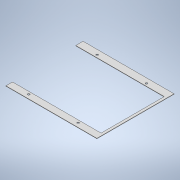
# Autodesk Inventor part: mainBody
Saved by Autodesk Inventor 2020.3 (Build 243373000, 373)
## iProperties
Created: 2021-03-06
Part Number: mainBody
Material: Generic
Document SubType Name: Modeling
Designer: allofus
Density: 1 g/cm^3
Appearance: Default
Author: allofus
Autodesk Inventor part; units mm, degrees
ref_plane "YZ Plane" through (0, 0, 0) normal (1, 0, 0) x (0, 1, 0)
ref_plane "XZ Plane" through (0, 0, 0) normal (0, 1, 0) x (-1, 0, 0)
ref_plane "XY Plane" through (0, 0, 0) normal (0, 0, 1) x (1, 0, 0)
sketch "Sketch1" plane through (0, 0, 0) normal (0, 1, 0) x (-1, 0, 0)
  circle A0 centre (0, 0) radius 2.5
  circle A1 centre (125, 0) radius 2.5
  circle A2 centre (125, 173) radius 2.5
  circle A3 centre (0, 173) radius 2.5
  line L0 (57.2025, 240.8064) -> (94.1768, 240.8064)
  line L1 (94.1768, 240.8064) -> (82.9725, 250.4701)
  line L2 (82.9725, 250.4701) -> (82.9725, 230.5824)
  line L3 (82.9725, 230.5824) -> (94.1768, 240.8064)
  line L4 (172.5, 183) -> (-57.5, 183)
  line L5 (-57.5, 183) -> (-57.5, -12)
  line L6 (-57.5, -12) -> (172.5, -12)
  line L7 (172.5, -12) -> (172.5, 183)
  line L8 (172.5, 6.4252) -> (-51.3543, 6.4252)
  line L9 (-51.3543, 6.4252) -> (-51.3543, 166.3217)
  line L10 (-51.3543, 166.3217) -> (172.5, 166.3217)
  line L11 (172.5, 166.3217) -> (172.5, 6.4252)
  dimension "d0" = 5
  dimension "d1" = 5
  dimension "d2" = 125
  dimension "d3" = 5
  dimension "d4" = 173
  dimension "d5" = 0
  dimension "d6" = 0
  dimension "d7" = 5
  dimension "d8" = 0
  dimension "d9" = 0
  dimension "d10" = 230
  dimension "d11" = 195
  dimension "d12" = 57.5
  dimension "d13" = 10
  constraints: 24 end point, 4 centre point, 4 parallel, 3 horizontal, 3 perpendicular, 1 coincident, 1 point on line
  measures "d0" diameter of A0
  measures "d1" diameter of A1
  measures "d2" distance of A1.centre point (0, 0)
  measures "d3" diameter of A2
  measures "d4" distance of A1.centre A2.centre
  measures "d5" horizontal distance of A1.centre A2.centre
  measures "d6" vertical distance of point (0, 0) A1.centre
  measures "d7" diameter of A3
  measures "d8" horizontal distance of point (0, 0) A3.centre
  measures "d9" vertical distance of A2.centre A3.centre
  measures "d10" distance of L6.end L5.end
  measures "d11" distance of L5.end L4.end
  measures "d12" horizontal distance of A3.centre L4.end
  measures "d13" vertical distance of A3.centre L4.end
extrude "Extrusion1" add sketch "Sketch1" along normal blind 1 contours L7 L10 L9 L8 L6 L5 L4
body "Solid1"
